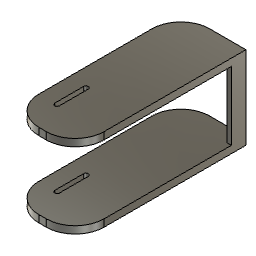
mounting bracket v3 (Autodesk Fusion 360 design; units mm, degrees)
Autodesk Fusion 360 part; units mm, degrees
note: some values were not read from the file. Set by a fixed rule: which sketch regions a step uses.
sketch "Sketch1" plane through (0, 0, 0) normal (0, 0, 1) x (1, 0, 0)
  line L0 (0, 0) -> (0, 25)
  line L1 (0, 0) -> (25, 0)
  line L2 (0, 25) -> (-3, 25)
  line L3 (25, 0) -> (25, -3)
  line L4 (25, -3) -> (-3, -3)
  line L5 (-3, 25) -> (-3, -3)
  dimension "d1" = 25
  dimension "d2" = 25
  dimension "d3" = 3
  dimension "d4" = 3
  constraint coincident L0.start L1.start
  constraint vertical L0
  constraint perpendicular L0 L1
  constraint perpendicular L0 L2
  constraint perpendicular L1 L3
  constraint perpendicular L3 L4
  measures "d1" distance of L0.start L0.end
  measures "d2" distance of L0.start L1.end
  measures "d3" distance of L0.end L2.end
  measures "d4" distance of L1.end L3.end
extrude "Extrude1" add sketch "Sketch1" along normal blind 20
sketch "Sketch2" plane through (0, 0, 20) normal (0, 0, 1) x (-1, 0, 0)
  line L0 (0, 0) -> (0, -25)
  line L1 (0, -25) -> (3, -25)
  line L2 (3, -25) -> (3, 3)
  line L3 (3, 3) -> (-25, 3)
  line L4 (-25, 3) -> (-25, 0)
  line L5 (-25, 0) -> (0, 0)
  line L6 (3, -25) -> (0, -25)
  line L7 (0, -25) -> (0, -15)
  line L8 (0, -15) -> (3, -15)
  line L9 (3, -15) -> (3, -25)
  line L10 (-25, 0) -> (-15, 0)
  line L11 (-15, 0) -> (-25, 0)
  line L12 (-25, 0) -> (-25, 3)
  line L13 (-25, 3) -> (-15, 3)
  line L14 (-15, 3) -> (-15, 0)
  dimension "d7" = 10
  constraint horizontal L6
  constraint vertical L7
  constraint horizontal L8
  constraint vertical L9
  constraint coincident L0 L7.end
  constraint coincident L1.end L2.start
  constraint coincident L4.end L5.start
  constraint perpendicular L4 L10
  constraint horizontal L11
  constraint vertical L12
  constraint horizontal L13
  constraint vertical L14
  constraint coincident L3.end L4.start
  measures "d7" distance of L4.end L10.end
extrude "Extrude2" add sketch "Sketch2" along normal blind 47.2 contours L0 L1 L2 L6 L7 L8 L9 | L3 L4 L5 L10 L11 L12 L13 L14
sketch "Sketch3" plane through (0, 0, 67.2) normal (0, 0, 1) x (-1, 0, 0)
  line L0 (3, -15) -> (0, -15)
  line L1 (0, -15) -> (0, -25)
  line L2 (0, -25) -> (3, -25)
  line L3 (3, -25) -> (3, -15)
  line L4 (3, -25) -> (3, 3)
  line L5 (3, 3) -> (-25, 3)
  line L6 (-25, 3) -> (-25, 0)
  line L7 (-25, 0) -> (0, 0)
  line L8 (0, 0) -> (0, -25)
  line L9 (3, -25) -> (0, -25)
  constraint coincident L2.end L3.start
  constraint perpendicular L2 L4
  constraint perpendicular L4 L5
  constraint perpendicular L5 L6
  constraint coincident L7.end L8.start
  constraint perpendicular L6 L7
  constraint coincident L1.end L2.start
extrude "Extrude3" add sketch "Sketch3" along normal blind 20
sketch "Sketch4" plane through (-3, 0, 0) normal (-1, 0, 0) x (0, -1, 0)
  line L0 (-25, 20) -> (-15, 20)
  line L1 (-15, 20) -> (-15, 67.2)
  line L2 (-15, 67.2) -> (3, 67.2)
  line L3 (3, 67.2) -> (3, 87.2)
  line L4 (3, 87.2) -> (-25, 87.2)
  line L5 (-25, 87.2) -> (-25, 20)
  line L6 (3, 67.2) -> (3, 72.2)
  line L7 (3, 20) -> (3, 15)
  line L8 (3, 15) -> (-25, 15)
  line L9 (-25, 15) -> (-25, 20)
  line L10 (-25, 20) -> (3, 20)
  line L11 (3, 20) -> (3, 15)
  line L12 (3, 72.2) -> (-25, 72.2)
  line L13 (-25, 72.2) -> (-25, 67.2)
  line L14 (-25, 67.2) -> (3, 67.2)
  line L15 (3, 67.2) -> (3, 72.2)
  dimension "d12" = 5
  dimension "d13" = 5
  constraint coincident L2.end L3.start
  constraint perpendicular L2 L6
  constraint vertical L7
  constraint horizontal L8
  constraint vertical L9
  constraint horizontal L10
  constraint vertical L11
  constraint coincident L0.start L5.end
  constraint horizontal L12
  constraint vertical L13
  constraint horizontal L14
  constraint vertical L15
  constraint coincident L5 L13.end
  measures "d12" distance of L2.end L6.end
  measures "d13" distance of L7.start L7.end
extrude "Extrude4" add sketch "Sketch4" along normal blind 45 contours L0 L7 L8 L9 L10 L11 | L2 L3 L5 L6 L12 L13 L14 L15
sketch "Sketch5" plane through (0, -3, 0) normal (0, -1, 0) x (1, 0, 0)
  line L0 (-3, 0) -> (25, 0)
  line L1 (25, 0) -> (25, 87.2)
  line L2 (25, 87.2) -> (-3, 87.2)
  line L3 (-3, 87.2) -> (-3, 72.2)
  line L4 (-3, 72.2) -> (-48, 72.2)
  line L5 (-48, 72.2) -> (-48, 67.2)
  line L6 (-48, 67.2) -> (15, 67.2)
  line L7 (15, 67.2) -> (15, 20)
  line L8 (15, 20) -> (-48, 20)
  line L9 (-48, 20) -> (-48, 15)
  line L10 (-48, 15) -> (-3, 15)
  line L11 (-3, 15) -> (-3, 0)
  line L12 (-3, 72.2) -> (-3, 15)
  line L13 (-48, 20) -> (-3, 20)
  line L14 (-3, 20) -> (-3, 15)
  line L15 (-3, 15) -> (-48, 15)
  line L16 (-48, 15) -> (-48, 20)
  line L17 (-48, 72.2) -> (-3, 72.2)
  line L18 (-3, 72.2) -> (-3, 67.2)
  line L19 (-3, 67.2) -> (-48, 67.2)
  line L20 (-48, 67.2) -> (-48, 72.2)
  dimension "d16" = 57.2
  constraint vertical L12
  constraint coincident L3.end L4.start
  constraint horizontal L13
  constraint vertical L14
  constraint horizontal L15
  constraint vertical L16
  constraint coincident L8.end L9.start
  constraint horizontal L17
  constraint vertical L18
  constraint horizontal L19
  constraint vertical L20
  constraint coincident L12 L18.end
  constraint coincident L6 L18.end
  constraint coincident L4.end L5.start
  measures "d16" distance of L3.end L10.end
extrude "Extrude5" add sketch "Sketch5" along normal blind 90 contours L8 L9 L10 L12 L13 L14 L15 L16 | L4 L5 L6 L12 L17 L18 L19 L20
sketch "Sketch6" plane through (0, 0, 72.2) normal (0, 0, 1) x (-1, 0, 0)
  line L0 (3, 3) -> (3, -25)
  line L1 (3, -25) -> (48, -25)
  line L2 (48, -25) -> (48, 93)
  line L3 (48, 93) -> (3, 93)
  line L4 (3, 93) -> (3, 3)
  line L5 (25.5, 93) -> (25.5, -25)
  line L6 (25.5, -25) -> (25.5, 17)
  circle A0 centre (25.5, 17) radius 1.6
  line L7 (25.5, 93) -> (25.5, 73)
  circle A1 centre (25.5, 73) radius 1.6
  line L8 (23.9056, 16.8667) -> (23.9, 72.9998)
  line L9 (27.1, 73) -> (27.1, 17)
  dimension "d19" = 42
  dimension "d20" = 3.2
  dimension "d21" = 20
  dimension "d22" = 3.2
  constraint midpoint L3 L5.start
  constraint midpoint L1 L5.end
  constraint perpendicular L1 L6
  constraint coincident L6.end A0.centre
  constraint perpendicular L3 L7
  constraint coincident L7.end A1.centre
  constraint coincident A0 L8.start
  constraint coincident A1 L8.end
  constraint tangent A1 L8
  constraint coincident A1 L9.start
  constraint coincident A0 L9.end
  constraint tangent A0 L9
  constraint parallel L7 L9
  measures "d19" distance of L5.end L6.end
  measures "d20" diameter of A0
  measures "d21" distance of L5.start L7.end
  measures "d22" diameter of A1
fillet "Fillet1" radius 20 6 edges at (-48, 25, 17.5) (-48, 25, 69.7) (-48, -93, 17.5) (-48, -93, 69.7) (-3, -93, 17.5) (-3, -93, 69.7)
extrude "Extrude7" cut 1 faces at (13.3333, 0, 80.5333) along direction (0, -1, 0) blind 10
extrude "Extrude8" cut 1 faces at (-2, 6.3333, 0) along direction (0, 0, 1) blind 15
extrude "Extrude9" cut 1 faces at (-1, 6.3333, 87.2) along direction (0, 0, -1) blind 15
extrude "Extrude10" add 1 faces at (-3, 21.6667, 35.7333) along direction (-1, 0, 0) blind 3
extrude "Extrude11" cut 1 faces at (0, 21.6667, 35.7333) along direction (-1, 0, 0) blind 3
sketch "Sketch7" plane through (0, 0, 15) normal (0, 0, -1) x (1, 0, 0)
  line L0 (-3, -25) -> (-3, 73)
  arc A0 (-3, 73) -> (-23, 93) centre (-23, 73) ccw
  line L1 (-23, 93) -> (-28, 93)
  arc A1 (-28, 93) -> (-48, 73) centre (-28, 73) ccw
  line L2 (-48, 73) -> (-48, -5)
  arc A2 (-48, -5) -> (-28, -25) centre (-28, -5) ccw
  line L3 (-28, -25) -> (-3, -25)
  line L4 (-25.5055, 73) -> (-35.5055, 73)
  circle A3 centre (-35.5055, 73) radius 1.6
  line L5 (-35.5055, 73) -> (-35.5055, 53)
  circle A4 centre (-35.5055, 53) radius 1.6
  line L6 (-35.5055, 53) -> (-33.9055, 53)
  line L7 (-33.9055, 53) -> (-33.9055, 73)
  line L8 (-33.9055, 73) -> (-35.5055, 73)
  line L9 (-35.5055, 73) -> (-35.5055, 53)
  line L10 (-37.1055, 53) -> (-37.1055, 73)
  dimension "d37" = 10
  dimension "d38" = 3.2
  dimension "d39" = 20
  dimension "d40" = 3.2
  constraint horizontal L4
  constraint coincident L4.end A3.centre
  constraint perpendicular L4 L5
  constraint coincident L5.end A4.centre
  constraint horizontal L6
  constraint vertical L7
  constraint horizontal L8
  constraint vertical L9
  constraint coincident A3 L7.end
  constraint coincident L4 L7.end
  constraint symmetric L6.end L9 L10.start
  constraint symmetric L7.end L9 L10.end
  measures "d37" distance of L4.start L4.end
  measures "d38" diameter of A3
  measures "d39" distance of L4.end L5.end
  measures "d40" diameter of A4
extrude "Extrude12" cut sketch "Sketch7" against normal blind 100 contours L4 A3 L5 L8 L9 | L4 A3 L5 L8 L9 | A3 L5 A4 L7 L9 | A3 L5 A4 L9 L10 | L5 A4 L6 L9 | L5 A4 L6 L9
named bodies: "Mounting Bracket"
